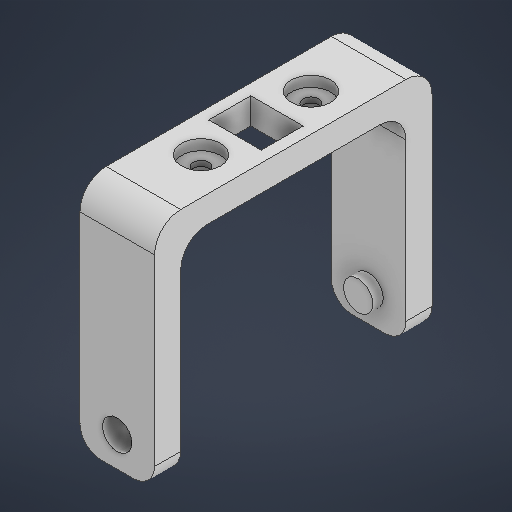
# Autodesk Inventor part: ruka_part spodni
Saved by Autodesk Inventor 2026 (Build 300175000, 175)
## iProperties
Created: 2025-04-11
Part Number: ruka_part spodni
Material: Generic
Document SubType Name: Modeling
Designer: janpa
Density: 1 g/cm^3
Appearance: Default
Author: janpa
Autodesk Inventor part; units mm, degrees
ref_plane "YZ Plane" through (0, 0, 0) normal (1, 0, 0) x (0, 1, 0)
ref_plane "XZ Plane" through (0, 0, 0) normal (0, 1, 0) x (-1, 0, 0)
ref_plane "XY Plane" through (0, 0, 0) normal (0, 0, 1) x (1, 0, 0)
sketch "Sketch2" plane through (0, 0, 0) normal (1, 0, 0) x (0, 1, 0)
  line L0 (0, 0) -> (39, 0)
  line L1 (44, -5) -> (44, -5)
  line L2 (34, -5) -> (0, -5)
  line L3 (0, -5) -> (0, 0)
  line L4 (39, -10) -> (39, -43)
  line L5 (44, -48) -> (44, -5)
  line L6 (0, -53) -> (0, -48)
  line L7 (39, -53) -> (0, -53)
  line L8 (0, -53) -> (0, -48)
  line L9 (0, -48) -> (34, -48)
  arc A0 (44, -5) -> (39, 0) centre (39, -5) ccw
  arc A1 (34, -48) -> (39, -43) centre (34, -43) ccw
  arc A2 (39, -10) -> (34, -5) centre (34, -10) ccw
  arc A3 (39, -53) -> (44, -48) centre (39, -48) ccw
  point P0 (44, 0)
  point P1 (0, -2.5)
  point P2 (0, -53)
  dimension "d12" = 44
  dimension "d14" = 5
  dimension "d17" = 5
  dimension "d18" = 39
  dimension "d19" = 5
  dimension "d42" = 43
  constraints: 20 end point, 8 point on circle, 8 tangent, 4 centre point, 4 parallel, 2 equal radius, 2 horizontal, 2 perpendicular, 2 point on line, 1 midpoint
  measures "d12" distance of L0.start point (44, 0)
  measures "d14" distance of L2.end L0.start
  measures "d17" distance of L6.end L7.end
  measures "d18" distance from line of point (0, -2.5) L4
  measures "d19" radius of A0
  measures "d42" distance between parallel lines of L9 L2
extrude "Extrusion2" add sketch "Sketch2" along normal blind 14.25
fillet "Fillet1" radius 4 4 edges at (14.25, 0, -2.5) (0, 0, -2.5) (14.25, 0, -50.5) (0, 0, -50.5)
sketch "Sketch3" plane through (0, 39, 0) normal (0, 0, 1) x (1, 0, 0)
  circle A0 centre (7.125, -33.3) radius 2.8
  line L0 (0, 0) -> (0, -35) projected
  line L1 (4, -39) -> (10.25, -39) projected
  point P0 (0, -39)
  point P1 (7.125, -39)
  dimension "d23" = 5.6
  dimension "d24" = 7.125
  dimension "d25" = 5.7
  constraints: 1 centre point, 1 midpoint
  measures "d23" diameter of A0
  measures "d24" distance from line of L0 A0.centre
  measures "d25" distance of point (7.125, -39) A0.centre
extrude "Extrusion3" cut sketch "Sketch3" against normal blind 11.4
sketch "Sketch7" plane through (0, 39, -43) normal (0, -1, 0) x (1, 0, 0)
  circle A0 centre (7.125, 27) radius 1.5
  circle A1 centre (7.125, 6) radius 1.5
  line L0 (0, 33) -> (0, 0) projected
  line L1 (14.25, 33) -> (14.25, 0) projected
  line L2 (0, 33) -> (14.25, 33) projected
  line L3 (0, 0) -> (14.25, 0) projected
  circle A2 centre (7.125, 27) radius 2.8
  circle A3 centre (7.125, 6) radius 2.8
  point P0 (0, 43)
  dimension "d30" = 3
  dimension "d31" = 3
  dimension "d32" = 7.125
  dimension "d33" = 7.125
  dimension "d34" = 6
  dimension "d35" = 6
  dimension "d36" = 5.6
  dimension "d37" = 5.6
  constraints: 4 centre point, 2 coincident
  measures "d30" diameter of A0
  measures "d31" diameter of A1
  measures "d32" distance from line of L0 A0.centre
  measures "d33" distance from line of L1 A1.centre
  measures "d34" distance from line of L2 A0.centre
  measures "d35" distance from line of L3 A1.centre
  measures "d36" diameter of A2
  measures "d37" diameter of A3
extrude "Extrusion5" cut sketch "Sketch7" against normal blind 8 contours A0 | A1
extrude "Extrusion6" cut sketch "Sketch7" against normal blind 2 contours A2 | A3
sketch "Sketch8" plane through (0, 34, -48) normal (0, 0, 1) x (1, 0, 0)
  circle A0 centre (7.125, -28.3) radius 2.8 projected
  circle A1 centre (7.125, -28.3) radius 2.8
  point P0 (0, -34)
  constraints: 1 centre point, 1 coincident
extrude "Extrusion7" add sketch "Sketch8" along normal blind 2
sketch "Sketch9" plane through (0, 44, -5) normal (0, 1, 0) x (1, 0, 0)
  circle A0 centre (7.125, 11) radius 1.5 projected
  circle A1 centre (7.125, 11) radius 3.75
  line L0 (0, 43) -> (0, 0) projected
  line L1 (0, 21.5) -> (1.5875, 21.5)
  circle A2 centre (7.125, 32) radius 3.75
  point P0 (0, -5)
  dimension "d46" = 7.5
  constraints: 2 centre point, 2 end point, 1 coincident, 1 horizontal, 1 midpoint, 1 symmetric about line, 1 other
  measures "d46" diameter of A1
extrude "Extrusion8" cut sketch "Sketch9" against normal blind 2 contours A0 | A1 | A2
sketch "Sketch10" plane through (0, 44, -5) normal (0, 1, 0) x (1, 0, 0)
  line L0 (2.125, 17.5) -> (12.125, 17.5)
  line L1 (12.125, 17.5) -> (12.125, 25.5)
  line L2 (12.125, 25.5) -> (2.125, 25.5)
  line L3 (2.125, 25.5) -> (2.125, 17.5)
  line L4 (0, 43) -> (0, 0) projected
  line L5 (14.25, 43) -> (14.25, 0) projected
  line L6 (0, 0) -> (14.25, 0) projected
  point P0 (0, -5)
  point P1 (0, 21.5)
  point P2 (14.25, 21.5)
  dimension "d49" = 10
  dimension "d50" = 8
  dimension "d51" = 2.125
  dimension "d52" = 2.125
  dimension "d53" = 17.5
  constraints: 8 end point, 2 midpoint, 2 parallel, 1 horizontal, 1 perpendicular
  measures "d49" distance of L2.end L1.end
  measures "d50" distance of L1.end L0.end
  measures "d51" distance from line of point (0, 21.5) L3
  measures "d52" distance from line of point (14.25, 21.5) L1
  measures "d53" distance between parallel lines of L6 L0
extrude "Extrusion9" cut sketch "Sketch10" against normal blind 50
body "Solid2"
